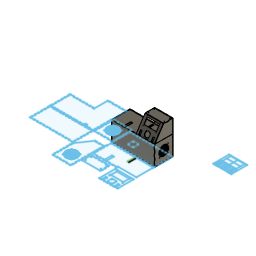
Music Inverntory Machine v29 (1) (Autodesk Fusion 360 design; units mm, degrees)
Autodesk Fusion 360 part; units mm, degrees
note: some values were not read from the file. Set by a fixed rule: which sketch regions a step uses.
(part 1 of 6)
sketch "300mm" plane through (0, 0, 0) normal (0, 0, 1) x (1, 0, 0)
  line L0 (3, 62.25) -> (0, 62.25)
  line L1 (164.25, 6) -> (186.75, 6)
  line L2 (0, 107.25) -> (0, 84.75)
  line L3 (119.25, 6) -> (141.75, 6)
  line L4 (303, 39.75) -> (306, 39.75)
  line L5 (0, 62.25) -> (0, 39.75)
  line L6 (306, 62.25) -> (303, 62.25)
  line L7 (303, 107.25) -> (303, 129.75)
  line L8 (96.75, 6) -> (96.75, 3)
  line L9 (306, 144) -> (276.75, 144)
  line L10 (0, 129.75) -> (3, 129.75)
  line L11 (306, 17.25) -> (303, 17.25)
  line L12 (276.75, 6) -> (276.75, 3)
  line L13 (0, 144) -> (0, 129.75)
  line L14 (51.75, 3) -> (74.25, 3)
  line L15 (231.75, 144) -> (231.75, 141)
  line L16 (74.25, 3) -> (74.25, 6)
  line L17 (306, 39.75) -> (306, 62.25)
  line L18 (231.75, 141) -> (209.25, 141)
  line L19 (0, 39.75) -> (3, 39.75)
  line L20 (186.75, 6) -> (186.75, 3)
  line L21 (96.75, 3) -> (119.25, 3)
  line L22 (74.25, 6) -> (96.75, 6)
  line L23 (254.25, 6) -> (276.75, 6)
  line L24 (0, 17.25) -> (0, 3)
  line L25 (303, 62.25) -> (303, 84.75)
  line L26 (306, 84.75) -> (306, 107.25)
  line L27 (306, 107.25) -> (303, 107.25)
  line L28 (3, 17.25) -> (0, 17.25)
  line L29 (254.25, 3) -> (254.25, 6)
  line L30 (141.75, 3) -> (164.25, 3)
  line L31 (303, 84.75) -> (306, 84.75)
  line L32 (0, 84.75) -> (3, 84.75)
  line L33 (231.75, 6) -> (231.75, 3)
  line L34 (276.75, 3) -> (299.25, 3)
  line L35 (306, 129.75) -> (306, 144)
  line L36 (303, 129.75) -> (306, 129.75)
  line L37 (276.75, 144) -> (276.75, 141)
  line L38 (254.25, 141) -> (254.25, 144)
  line L39 (209.25, 141) -> (209.25, 144)
  line L40 (276.75, 141) -> (254.25, 141)
  line L41 (51.75, 6) -> (51.75, 3)
  line L42 (254.25, 144) -> (231.75, 144)
  line L43 (0, 3) -> (29.25, 3)
  line L44 (231.75, 3) -> (254.25, 3)
  line L45 (3, 107.25) -> (0, 107.25)
  line L46 (209.25, 144) -> (186.75, 144)
  line L47 (209.25, 6) -> (231.75, 6)
  line L48 (29.25, 3) -> (29.25, 6)
  line L49 (3, 129.75) -> (3, 107.25)
  line L50 (141.75, 6) -> (141.75, 3)
  line L51 (299.25, 3) -> (306, 3)
  line L52 (303, 17.25) -> (303, 39.75)
  line L53 (209.25, 3) -> (209.25, 6)
  line L54 (119.25, 3) -> (119.25, 6)
  line L55 (3, 84.75) -> (3, 62.25)
  line L56 (29.25, 6) -> (51.75, 6)
  line L57 (306, 3) -> (306, 17.25)
  line L58 (164.25, 3) -> (164.25, 6)
  line L59 (186.75, 3) -> (209.25, 3)
  line L60 (3, 39.75) -> (3, 17.25)
  line L61 (51.75, 144) -> (51.75, 141)
  line L62 (96.75, 144) -> (96.75, 141)
  line L63 (74.25, 144) -> (51.75, 144)
  line L64 (141.75, 144) -> (141.75, 141)
  line L65 (186.75, 141) -> (164.25, 141)
  line L66 (29.25, 144) -> (6.75, 144)
  line L67 (96.75, 141) -> (74.25, 141)
  line L68 (6.75, 144) -> (0, 144)
  line L69 (74.25, 141) -> (74.25, 144)
  line L70 (164.25, 144) -> (141.75, 144)
  line L71 (119.25, 141) -> (119.25, 144)
  line L72 (141.75, 141) -> (119.25, 141)
  line L73 (119.25, 144) -> (96.75, 144)
  line L74 (51.75, 141) -> (29.25, 141)
  line L75 (186.75, 144) -> (186.75, 141)
  line L76 (164.25, 141) -> (164.25, 144)
  line L77 (29.25, 141) -> (29.25, 144)
  line L78 (441, -20.25) -> (438, -20.25)
  line L79 (441, -42.75) -> (441, -20.25)
  line L80 (408.75, 90.147) -> (408.75, 87.147)
  line L81 (438, -42.75) -> (441, -42.75)
  line L82 (438, -147) -> (438, -132.75)
  line L83 (312, -6) -> (312, -20.25)
  line L84 (438, 90.147) -> (408.75, 90.147)
  line L85 (431.25, -147) -> (438, -147)
  line L86 (309, -87.75) -> (312, -87.75)
  line L87 (312, -42.75) -> (312, -65.25)
  line L88 (312, -87.75) -> (312, -110.25)
  line L89 (441, -132.75) -> (441, -110.25)
  line L90 (309, -42.75) -> (312, -42.75)
  line L91 (312, -65.25) -> (309, -65.25)
  line L92 (438, -20.25) -> (438, 90.147)
  line L93 (363.75, -144) -> (363.75, -147)
  line L94 (408.75, 87.147) -> (386.25, 87.147)
  line L95 (341.25, -144) -> (363.75, -144)
  line L96 (309, -110.25) -> (309, -132.75)
  line L97 (309, -132.75) -> (312, -132.75)
  line L98 (441, -87.75) -> (441, -65.25)
  line L99 (408.75, -147) -> (431.25, -147)
  line L100 (312, -147) -> (341.25, -147)
  line L101 (309, -65.25) -> (309, -87.75)
  line L102 (438, -132.75) -> (441, -132.75)
  line L103 (312, -20.25) -> (309, -20.25)
  line L104 (408.75, -144) -> (408.75, -147)
  line L105 (341.25, -147) -> (341.25, -144)
  line L106 (386.25, 87.147) -> (386.25, 90.147)
  line L107 (312, -132.75) -> (312, -147)
  line L108 (441, -65.25) -> (438, -65.25)
  line L109 (312, -110.25) -> (309, -110.25)
  line L110 (363.75, -147) -> (386.25, -147)
  line L111 (438, -87.75) -> (441, -87.75)
  line L112 (438, -110.25) -> (438, -87.75)
  line L113 (441, -110.25) -> (438, -110.25)
  line L114 (386.25, -147) -> (386.25, -144)
  line L115 (309, -20.25) -> (309, -42.75)
  line L116 (386.25, -144) -> (408.75, -144)
  line L117 (438, -65.25) -> (438, -42.75)
  line L118 (447, 6) -> (473.25, 6)
  line L119 (447, 57.75) -> (444, 57.75)
  line L120 (447, 80.25) -> (447, 57.75)
  line L121 (473.25, 6) -> (473.25, 3)
  line L122 (585.75, 3) -> (585.75, 6)
  line L123 (608.25, 6) -> (608.25, 3)
  line L124 (447, 35.25) -> (447, 12.75)
  line L125 (540.75, 6) -> (563.25, 6)
  line L126 (447, 102.75) -> (444, 102.75)
  line L127 (495.75, 6) -> (518.25, 6)
  line L128 (563.25, 132) -> (540.75, 132)
  line L129 (608.25, 132) -> (585.75, 132)
  line L130 (540.75, 132) -> (540.75, 135)
  line L131 (585.75, 132) -> (585.75, 135)
  line L132 (747, 132) -> (617.8, 132)
  line L133 (747, 125.25) -> (747, 132)
  line L134 (447, 132) -> (447, 102.75)
  line L135 (495.75, 3) -> (495.75, 6)
  line L136 (518.25, 135) -> (518.25, 132)
  line L137 (444, 35.25) -> (447, 35.25)
  line L138 (444, 102.75) -> (444, 80.25)
  line L139 (563.25, 3) -> (585.75, 3)
  line L140 (447, 12.75) -> (447, 6)
  line L141 (563.25, 6) -> (563.25, 3)
  line L142 (518.25, 6) -> (518.25, 3)
  line L143 (585.75, 6) -> (608.25, 6)
  line L144 (540.75, 3) -> (540.75, 6)
  line L145 (608.25, 135) -> (608.25, 132)
  line L146 (473.25, 3) -> (495.75, 3)
  line L147 (747, 12) -> (747, 125.25)
  line L148 (518.25, 3) -> (540.75, 3)
  line L149 (444, 57.75) -> (444, 35.25)
  line L150 (444, 80.25) -> (447, 80.25)
  line L151 (518.25, 132) -> (495.75, 132)
  line L152 (473.25, 132) -> (450.75, 132)
  line L153 (495.75, 132) -> (495.75, 135)
  line L154 (473.25, 135) -> (473.25, 132)
  line L155 (563.25, 135) -> (563.25, 132)
  line L156 (450.75, 132) -> (447, 132)
  line L157 (540.75, 135) -> (518.25, 135)
  line L158 (585.75, 135) -> (563.25, 135)
  line L159 (495.75, 135) -> (473.25, 135)
  line L160 (29.25, 150) -> (51.75, 150)
  line L161 (51.75, 150) -> (51.75, 147)
  line L162 (276.75, 150) -> (276.75, 147)
  line L163 (0, 161.25) -> (0, 147)
  line L164 (29.25, 147) -> (29.25, 150)
  line L165 (96.75, 147) -> (119.25, 147)
  line L166 (51.75, 147) -> (74.25, 147)
  line L167 (3, 206.25) -> (0, 206.25)
  line L168 (209.25, 147) -> (209.25, 150)
  line L169 (119.25, 147) -> (119.25, 150)
  line L170 (3, 251.25) -> (0, 251.25)
  line L171 (231.75, 147) -> (254.25, 147)
  line L172 (209.25, 150) -> (231.75, 150)
  line L173 (3, 161.25) -> (0, 161.25)
  line L174 (231.75, 150) -> (231.75, 147)
  line L175 (0, 206.25) -> (0, 183.75)
  line L176 (254.25, 147) -> (254.25, 150)
  line L177 (0, 183.75) -> (3, 183.75)
  line L178 (3, 273.75) -> (3, 251.25)
  line L179 (74.25, 147) -> (74.25, 150)
  line L180 (0, 147) -> (29.25, 147)
  line L181 (119.25, 150) -> (141.75, 150)
  line L182 (164.25, 147) -> (164.25, 150)
  line L183 (3, 228.75) -> (3, 206.25)
  line L184 (164.25, 150) -> (186.75, 150)
  line L185 (186.75, 147) -> (209.25, 147)
  line L186 (0, 273.75) -> (3, 273.75)
  line L187 (303, 206.25) -> (303, 228.75)
  line L188 (141.75, 150) -> (141.75, 147)
  line L189 (306, 206.25) -> (303, 206.25)
  line L190 (96.75, 150) -> (96.75, 147)
  line L191 (276.75, 384.147) -> (276.75, 381.147)
  line L192 (299.25, 147) -> (306, 147)
  line L193 (141.75, 147) -> (164.25, 147)
  line L194 (0, 228.75) -> (3, 228.75)
  line L195 (0, 288) -> (0, 273.75)
  line L196 (74.25, 150) -> (96.75, 150)
  line L197 (186.75, 150) -> (186.75, 147)
  line L198 (254.25, 150) -> (276.75, 150)
  line L199 (276.75, 147) -> (299.25, 147)
  line L200 (0, 251.25) -> (0, 228.75)
  line L201 (3, 183.75) -> (3, 161.25)
  line L202 (231.75, 381.147) -> (209.25, 381.147)
  line L203 (164.25, 288) -> (141.75, 288)
  line L204 (306, 273.75) -> (306, 384.147)
  line L205 (96.75, 288) -> (96.75, 285)
  line L206 (51.75, 285) -> (29.25, 285)
  line L207 (303, 251.25) -> (303, 273.75)
  line L208 (141.75, 285) -> (119.25, 285)
  line L209 (186.75, 384.147) -> (186.75, 381.147)
  line L210 (306, 183.75) -> (306, 206.25)
  line L211 (306, 384.147) -> (276.75, 384.147)
  line L212 (141.75, 288) -> (141.75, 285)
  line L213 (254.25, 381.147) -> (254.25, 384.147)
  line L214 (276.75, 381.147) -> (254.25, 381.147)
  line L215 (254.25, 384.147) -> (231.75, 384.147)
  line L216 (6.75, 288) -> (0, 288)
  line L217 (231.75, 384.147) -> (231.75, 381.147)
  line L218 (306, 228.75) -> (306, 251.25)
  line L219 (303, 228.75) -> (306, 228.75)
  line L220 (29.25, 288) -> (6.75, 288)
  line L221 (29.25, 285) -> (29.25, 288)
  line L222 (164.25, 285) -> (164.25, 288)
  line L223 (96.75, 285) -> (74.25, 285)
  line L224 (119.25, 285) -> (119.25, 288)
  line L225 (306, 251.25) -> (303, 251.25)
  line L226 (119.25, 288) -> (96.75, 288)
  line L227 (74.25, 288) -> (51.75, 288)
  line L228 (209.25, 384.147) -> (186.75, 384.147)
  line L229 (306, 161.25) -> (303, 161.25)
  line L230 (209.25, 381.147) -> (209.25, 384.147)
  line L231 (303, 161.25) -> (303, 183.75)
  line L232 (303, 273.75) -> (306, 273.75)
  line L233 (173.8, 285) -> (164.25, 285)
  line L234 (303, 183.75) -> (306, 183.75)
  line L235 (306, 147) -> (306, 161.25)
  line L236 (51.75, 288) -> (51.75, 285)
  line L237 (74.25, 285) -> (74.25, 288)
  line L238 (309, 161.25) -> (312, 161.25)
  line L239 (386.25, 285) -> (386.25, 288)
  line L240 (312, 206.25) -> (312, 183.75)
  line L241 (309, 228.75) -> (309, 206.25)
  line L242 (309, 183.75) -> (309, 161.25)
  line L243 (341.25, 150) -> (363.75, 150)
  line L244 (386.25, 147) -> (386.25, 150)
  line L245 (441, 183.75) -> (438, 183.75)
  line L246 (341.25, 285) -> (341.25, 288)
  line L247 (438, 288) -> (408.75, 288)
  line L248 (341.25, 288) -> (318.75, 288)
  line L249 (438, 228.75) -> (438, 251.25)
  line L250 (386.25, 150) -> (408.75, 150)
  line L251 (312, 251.25) -> (312, 228.75)
  line L252 (309, 273.75) -> (309, 251.25)
  line L253 (309, 206.25) -> (312, 206.25)
  line L254 (438, 183.75) -> (438, 206.25)
  line L255 (408.75, 288) -> (408.75, 285)
  line L256 (438, 273.75) -> (438, 288)
  line L257 (363.75, 285) -> (341.25, 285)
  line L258 (312, 183.75) -> (309, 183.75)
  line L259 (312, 228.75) -> (309, 228.75)
  line L260 (312, 161.25) -> (312, 147)
  line L261 (309, 251.25) -> (312, 251.25)
  line L262 (408.75, 285) -> (386.25, 285)
  line L263 (312, 273.75) -> (309, 273.75)
  line L264 (363.75, 147) -> (386.25, 147)
  line L265 (318.75, 288) -> (312, 288)
  line L266 (363.75, 288) -> (363.75, 285)
  line L267 (441, 251.25) -> (441, 273.75)
  line L268 (441, 161.25) -> (441, 183.75)
  line L269 (386.25, 288) -> (363.75, 288)
  line L270 (341.25, 147) -> (341.25, 150)
  line L271 (438, 206.25) -> (441, 206.25)
  line L272 (438, 147) -> (438, 161.25)
  line L273 (431.25, 147) -> (438, 147)
  line L274 (438, 251.25) -> (441, 251.25)
  line L275 (438, 161.25) -> (441, 161.25)
  line L276 (312, 147) -> (341.25, 147)
  line L277 (363.75, 150) -> (363.75, 147)
  line L278 (408.75, 150) -> (408.75, 147)
  line L279 (441, 273.75) -> (438, 273.75)
  line L280 (312, 288) -> (312, 273.75)
  line L281 (408.75, 147) -> (431.25, 147)
  line L282 (441, 206.25) -> (441, 228.75)
  line L283 (441, 228.75) -> (438, 228.75)
  line L284 (447, 141) -> (473.25, 141)
  line L285 (585.75, 138) -> (585.75, 141)
  line L286 (698.25, 141) -> (698.25, 138)
  line L287 (447, 192.75) -> (444, 192.75)
  line L288 (608.25, 141) -> (608.25, 138)
  line L289 (447, 267) -> (447, 237.75)
  line L290 (444, 170.25) -> (447, 170.25)
  line L291 (495.75, 138) -> (495.75, 141)
  line L292 (585.75, 141) -> (608.25, 141)
  line L293 (747, 170.25) -> (750, 170.25)
  line L294 (675.75, 141) -> (698.25, 141)
  line L295 (750, 170.25) -> (750, 192.75)
  line L296 (743.25, 141) -> (747, 141)
  line L297 (608.25, 138) -> (630.75, 138)
  line L298 (447, 147.75) -> (447, 141)
  line L299 (747, 141) -> (747, 170.25)
  line L300 (630.75, 141) -> (653.25, 141)
  line L301 (563.25, 138) -> (585.75, 138)
  line L302 (447, 215.25) -> (447, 192.75)
  line L303 (675.75, 138) -> (675.75, 141)
  line L304 (518.25, 138) -> (540.75, 138)
  line L305 (495.75, 141) -> (518.25, 141)
  line L306 (653.25, 141) -> (653.25, 138)
  line L307 (447, 170.25) -> (447, 147.75)
  line L308 (698.25, 138) -> (720.75, 138)
  line L309 (444, 215.25) -> (447, 215.25)
  line L310 (447, 237.75) -> (444, 237.75)
  line L311 (540.75, 138) -> (540.75, 141)
  line L312 (630.75, 138) -> (630.75, 141)
  line L313 (653.25, 138) -> (675.75, 138)
  line L314 (720.75, 138) -> (720.75, 141)
  line L315 (518.25, 141) -> (518.25, 138)
  line L316 (720.75, 141) -> (743.25, 141)
  line L317 (444, 192.75) -> (444, 170.25)
  line L318 (608.25, 270) -> (608.25, 267)
  line L319 (720.75, 270) -> (698.25, 270)
  line L320 (630.75, 270) -> (608.25, 270)
  line L321 (563.25, 267) -> (540.75, 267)
  line L322 (747, 267) -> (720.75, 267)
  line L323 (747, 237.75) -> (747, 260.25)
  line L324 (675.75, 267) -> (675.75, 270)
  line L325 (495.75, 270) -> (473.25, 270)
  line L326 (585.75, 267) -> (585.75, 270)
  line L327 (630.75, 267) -> (630.75, 270)
  line L328 (750, 215.25) -> (750, 237.75)
  line L329 (747, 260.25) -> (747, 267)
  line L330 (720.75, 267) -> (720.75, 270)
  line L331 (518.25, 270) -> (518.25, 267)
  line L332 (540.75, 270) -> (518.25, 270)
  line L333 (747, 215.25) -> (750, 215.25)
  line L334 (675.75, 270) -> (653.25, 270)
  line L335 (750, 192.75) -> (747, 192.75)
  line L336 (698.25, 270) -> (698.25, 267)
  line L337 (473.25, 141) -> (473.25, 138)
  line L338 (495.75, 267) -> (495.75, 270)
  line L339 (540.75, 267) -> (540.75, 270)
  line L340 (540.75, 141) -> (563.25, 141)
  line L341 (563.25, 270) -> (563.25, 267)
  line L342 (653.25, 267) -> (630.75, 267)
  line L343 (747, 192.75) -> (747, 215.25)
  line L344 (563.25, 141) -> (563.25, 138)
  line L345 (473.25, 267) -> (450.75, 267)
  line L346 (750, 237.75) -> (747, 237.75)
  line L347 (698.25, 267) -> (675.75, 267)
  line L348 (585.75, 270) -> (563.25, 270)
  line L349 (450.75, 267) -> (447, 267)
  line L350 (653.25, 270) -> (653.25, 267)
  line L351 (473.25, 138) -> (495.75, 138)
  line L352 (608.25, 267) -> (585.75, 267)
  line L353 (518.25, 267) -> (495.75, 267)
  line L354 (473.25, 270) -> (473.25, 267)
  line L355 (444, 237.75) -> (444, 215.25)
  line L356 (396.25, 205.4178) -> (394.25, 206.5725)
  line L357 (397.75, 203.1084) -> (399.75, 201.9537)
  line L358 (401.75, 203.1084) -> (401.75, 205.4178)
  line L359 (399, 200.6547) -> (397, 201.8094)
  line L360 (396.25, 203.1084) -> (396.25, 205.4178)
  line L361 (401.75, 205.4178) -> (399.75, 206.5725)
  line L362 (395, 198.3453) -> (397, 197.1906)
  line L363 (401.75, 196.4178) -> (399.75, 197.5725)
  line L364 (397.75, 196.4178) -> (397.75, 194.1084)
  line L365 (397.75, 196.4178) -> (397.75, 194.1084)
  arc A0 (400.2057, 193.2169) -> (401.75, 194.9293) centre (375, 217.5) ccw
  line L366 (397, 197.1906) -> (399, 198.3453)
  line L367 (397.75, 194.1084) -> (399.75, 192.9537)
  line L368 (396.25, 196.4178) -> (394.25, 197.5725)
  line L369 (396.25, 196.4178) -> (394.25, 197.5725)
  line L370 (401.75, 194.9293) -> (401.75, 196.4178)
  line L371 (399.75, 192.9537) -> (400.2057, 193.2169)
  arc A1 (400.2057, 193.2169) -> (401.75, 194.9293) centre (375, 217.5) ccw
  line L372 (396.25, 194.1084) -> (396.25, 196.4178)
  line L373 (396.25, 194.1084) -> (396.25, 196.4178)
  line L374 (401.75, 196.4178) -> (399.75, 197.5725)
  line L375 (397.75, 194.1084) -> (399.75, 192.9537)
  line L376 (399.75, 192.9537) -> (400.2057, 193.2169)
  line L377 (399.75, 197.5725) -> (397.75, 196.4178)
  line L378 (401.75, 194.9293) -> (401.75, 196.4178)
  line L379 (395, 198.3453) -> (397, 197.1906)
  line L380 (399.75, 197.5725) -> (397.75, 196.4178)
  line L381 (397, 197.1906) -> (399, 198.3453)
  line L382 (394.25, 192.9537) -> (396.25, 194.1084)
  line L383 (394.25, 192.9537) -> (396.25, 194.1084)
  line L384 (375, 188.1906) -> (377, 189.3453)
  line L385 (389.5, 191.6547) -> (389.5, 189.3453)
  arc A2 (395.442, 189.0901) -> (398.7552, 191.7961) centre (375, 217.5) ccw
  line L386 (395, 189.3453) -> (395.442, 189.0901)
  line L387 (395, 191.6547) -> (395, 189.3453)
  arc A3 (395.442, 189.0901) -> (398.7552, 191.7961) centre (375, 217.5) ccw
  line L388 (395, 191.6547) -> (395, 189.3453)
  line L389 (395, 189.3453) -> (395.442, 189.0901)
  line L390 (396.25, 212.1084) -> (396.25, 214.4178)
  line L391 (397.75, 214.4178) -> (397.75, 212.1084)
  line L392 (377, 236.6547) -> (375, 237.8094)
  line L393 (395, 216.3453) -> (397, 215.1906)
  line L394 (399.75, 210.9537) -> (401.75, 212.1084)
  line L395 (375, 206.1906) -> (377, 207.3453)
  line L396 (399, 209.6547) -> (397, 210.8094)
  line L397 (397.75, 212.1084) -> (399.75, 210.9537)
  line L398 (399, 209.6547) -> (397, 210.8094)
  line L399 (397.75, 212.1084) -> (399.75, 210.9537)
  line L400 (396.25, 214.4178) -> (394.25, 215.5725)
  line L401 (375, 197.1906) -> (377, 198.3453)
  line L402 (397.75, 214.4178) -> (397.75, 212.1084)
  line L403 (375, 206.1906) -> (377, 207.3453)
  line L404 (401.75, 212.1084) -> (401.75, 214.4178)
  line L405 (375, 224.1906) -> (377, 225.3453)
  line L406 (394.25, 210.9537) -> (396.25, 212.1084)
  arc A4 (377, 252.4428) -> (373, 252.4428) centre (375, 217.5) ccw
  line L407 (375, 215.1906) -> (377, 216.3453)
  line L408 (377, 209.6547) -> (375, 210.8094)
  line L409 (375, 233.1906) -> (377, 234.3453)
  line L410 (399.75, 210.9537) -> (401.75, 212.1084)
  line L411 (377, 182.6547) -> (375, 183.8094)
  line L412 (375, 215.1906) -> (377, 216.3453)
  line L413 (375, 251.1906) -> (377, 252.3453)
  line L414 (401.75, 214.4178) -> (399.75, 215.5725)
  line L415 (395, 216.3453) -> (397, 215.1906)
  line L416 (377, 245.6547) -> (375, 246.8094)
  line L417 (401.75, 214.4178) -> (399.75, 215.5725)
  line L418 (396.25, 214.4178) -> (394.25, 215.5725)
  line L419 (396.25, 212.1084) -> (396.25, 214.4178)
  line L420 (375, 188.1906) -> (377, 189.3453)
  line L421 (375, 224.1906) -> (377, 225.3453)
  line L422 (377, 200.6547) -> (375, 201.8094)
  line L423 (375, 251.1906) -> (377, 252.3453)
  line L424 (397, 215.1906) -> (399, 216.3453)
  line L425 (377, 191.6547) -> (375, 192.8094)
  line L426 (377, 182.6547) -> (375, 183.8094)
  line L427 (377, 236.6547) -> (375, 237.8094)
  line L428 (397, 210.8094) -> (395, 209.6547)
  line L429 (377, 227.6547) -> (375, 228.8094)
  line L430 (375, 197.1906) -> (377, 198.3453)
  line L431 (377, 200.6547) -> (375, 201.8094)
  line L432 (377, 209.6547) -> (375, 210.8094)
  line L433 (398.7552, 191.7961) -> (397, 192.8094)
  line L434 (377, 191.6547) -> (375, 192.8094)
  line L435 (401.75, 223.4178) -> (399.75, 224.5725)
  line L436 (394.25, 197.5725) -> (392.25, 196.4178)
  arc A5 (342.75, 203.9008) -> (343.2193, 202.8375) centre (375, 217.5) ccw
  line L437 (391.5, 215.1906) -> (393.5, 216.3453)
  line L438 (348.25, 205.4178) -> (348.25, 203.1084)
  line L439 (386, 192.8094) -> (384, 191.6547)
  line L440 (368.75, 203.1084) -> (368.75, 205.4178)
  line L441 (375, 242.1906) -> (377, 243.3453)
  line L442 (353.75, 205.4178) -> (353.75, 203.1084)
  line L443 (377, 227.6547) -> (375, 228.8094)
  line L444 (399.75, 215.5725) -> (397.75, 214.4178)
  line L445 (380.5, 192.8094) -> (378.5, 191.6547)
  line L446 (377, 218.6547) -> (375, 219.8094)
  line L447 (397, 215.1906) -> (399, 216.3453)
  line L448 (346.75, 203.1084) -> (346.75, 205.4178)
  line L449 (386, 192.8094) -> (384, 191.6547)
  line L450 (382.5, 191.6547) -> (380.5, 192.8094)
  line L451 (399.75, 215.5725) -> (397.75, 214.4178)
  line L452 (391.5, 192.8094) -> (389.5, 191.6547)
  arc A6 (342.75, 203.9008) -> (343.2193, 202.8375) centre (375, 217.5) ccw
  line L453 (363.25, 203.1084) -> (363.25, 205.4178)
  line L454 (348.25, 205.4178) -> (348.25, 203.1084)
  line L455 (359.25, 205.4178) -> (359.25, 203.1084)
  line L456 (394.25, 210.9537) -> (396.25, 212.1084)
  line L457 (353.75, 205.4178) -> (353.75, 203.1084)
  line L458 (397, 192.8094) -> (395, 191.6547)
  line L459 (377, 245.6547) -> (375, 246.8094)
  line L460 (352.25, 203.1084) -> (352.25, 205.4178)
  line L461 (393.5, 191.6547) -> (391.5, 192.8094)
  line L462 (391.5, 192.8094) -> (389.5, 191.6547)
  line L463 (382.5, 191.6547) -> (380.5, 192.8094)
  line L464 (395, 225.3453) -> (397, 224.1906)
  line L465 (399, 218.6547) -> (397, 219.8094)
  line L466 (398.7552, 191.7961) -> (397, 192.8094)
  line L467 (397, 210.8094) -> (395, 209.6547)
  line L468 (388, 191.6547) -> (386, 192.8094)
  line L469 (401.75, 212.1084) -> (401.75, 214.4178)
  line L470 (380.5, 192.8094) -> (378.5, 191.6547)
  arc A7 (373, 182.5572) -> (377, 182.5572) centre (375, 217.5) ccw
  line L471 (396.25, 221.1084) -> (396.25, 223.4178)
  line L472 (357.75, 203.1084) -> (357.75, 205.4178)
  line L473 (377, 218.6547) -> (375, 219.8094)
  line L474 (357.75, 203.1084) -> (357.75, 205.4178)
  line L475 (397, 192.8094) -> (395, 191.6547)
  line L476 (346.75, 203.1084) -> (346.75, 205.4178)
  line L477 (399, 218.6547) -> (397, 219.8094)
  line L478 (374.25, 203.1084) -> (374.25, 205.4178)
  line L479 (397, 219.8094) -> (395, 218.6547)
  line L480 (370.25, 205.4178) -> (370.25, 203.1084)
  line L481 (364.75, 205.4178) -> (364.75, 203.1084)
  line L482 (396.25, 221.1084) -> (396.25, 223.4178)
  line L483 (359.25, 205.4178) -> (359.25, 203.1084)
  arc A8 (373, 182.5572) -> (377, 182.5572) centre (375, 217.5) ccw
  line L484 (393.5, 191.6547) -> (391.5, 192.8094)
  line L485 (388, 191.6547) -> (386, 192.8094)
  line L486 (352.25, 203.1084) -> (352.25, 205.4178)
  line L487 (364.75, 205.4178) -> (364.75, 203.1084)
  line L488 (368.75, 203.1084) -> (368.75, 205.4178)
  line L489 (397.75, 223.4178) -> (397.75, 221.1084)
  line L490 (363.25, 203.1084) -> (363.25, 205.4178)
  line L491 (401.75, 223.4178) -> (399.75, 224.5725)
  line L492 (394.25, 219.9537) -> (396.25, 221.1084)
  line L493 (363.25, 187.4178) -> (361.25, 188.5725)
  line L494 (359.25, 194.1084) -> (361.25, 192.9537)
  line L495 (361.25, 197.5725) -> (359.25, 196.4178)
  line L496 (392.25, 203.1084) -> (394.25, 201.9537)
  line L497 (344.75, 201.9537) -> (346.75, 203.1084)
  line L498 (370.25, 205.4178) -> (370.25, 203.1084)
  line L499 (347.5, 197.1906) -> (349.5, 198.3453)
  line L500 (344.75, 215.5725) -> (342.75, 214.4178)
  line L501 (391.5, 206.1906) -> (393.5, 207.3453)
  line L502 (347.5, 197.1906) -> (349.5, 198.3453)
  line L503 (392.25, 239.1084) -> (394.25, 237.9537)
  line L504 (392.25, 221.1084) -> (394.25, 219.9537)
  line L505 (394.25, 215.5725) -> (392.25, 214.4178)
  line L506 (347.5, 201.8094) -> (345.5, 200.6547)
  line L507 (349.5, 200.6547) -> (347.5, 201.8094)
  line L508 (374.25, 203.1084) -> (374.25, 205.4178)
  line L509 (344.75, 233.5725) -> (343.5641, 232.8879)
  line L510 (392.25, 203.1084) -> (394.25, 201.9537)
  line L511 (342.75, 212.1084) -> (344.75, 210.9537)
  line L512 (342.75, 221.1084) -> (344.75, 219.9537)
  line L513 (344.75, 206.5725) -> (342.75, 205.4178)
  line L514 (401.75, 221.1084) -> (401.75, 223.4178)
  line L515 (393.5, 209.6547) -> (391.5, 210.8094)
  line L516 (344.75, 224.5725) -> (342.75, 223.4178)
  line L517 (397, 224.1906) -> (399, 225.3453)
  line L518 (399.75, 224.5725) -> (397.75, 223.4178)
  line L519 (397.75, 223.4178) -> (397.75, 221.1084)
  line L520 (391.5, 233.1906) -> (393.5, 234.3453)
  line L521 (345.8335, 198.1527) -> (347.5, 197.1906)
  line L522 (345.8335, 198.1527) -> (347.5, 197.1906)
  line L523 (391.5, 242.1906) -> (393.5, 243.3453)
  line L524 (391.5, 224.1906) -> (393.5, 225.3453)
  line L525 (399.75, 219.9537) -> (401.75, 221.1084)
  line L526 (391.5, 224.1906) -> (393.5, 225.3453)
  line L527 (392.25, 221.1084) -> (394.25, 219.9537)
  line L528 (342.75, 230.1084) -> (344.75, 228.9537)
  line L529 (396.25, 223.4178) -> (394.25, 224.5725)
  line L530 (393.5, 200.6547) -> (391.5, 201.8094)
  line L531 (342.75, 212.1084) -> (344.75, 210.9537)
  line L532 (347.5, 201.8094) -> (345.5, 200.6547)
  line L533 (397, 219.8094) -> (395, 218.6547)
  line L534 (397.75, 221.1084) -> (399.75, 219.9537)
  line L535 (396.25, 223.4178) -> (394.25, 224.5725)
  line L536 (391.5, 233.1906) -> (393.5, 234.3453)
  line L537 (344.75, 215.5725) -> (342.75, 214.4178)
  line L538 (397.75, 221.1084) -> (399.75, 219.9537)
  line L539 (344.75, 206.5725) -> (342.75, 205.4178)
  line L540 (394.25, 219.9537) -> (396.25, 221.1084)
  line L541 (344.75, 224.5725) -> (342.75, 223.4178)
  line L542 (349.5, 200.6547) -> (347.5, 201.8094)
  line L543 (342.75, 230.1084) -> (344.75, 228.9537)
  line L544 (393.5, 209.6547) -> (391.5, 210.8094)
  line L545 (395, 225.3453) -> (397, 224.1906)
  line L546 (394.25, 242.5725) -> (392.25, 241.4178)
  line L547 (401.75, 221.1084) -> (401.75, 223.4178)
  line L548 (393.5, 245.6547) -> (391.5, 246.8094)
  line L549 (393.5, 216.3453) -> (393.5, 218.6547)
  line L550 (399, 216.3453) -> (399, 218.6547)
  line L551 (363.25, 214.4178) -> (361.25, 215.5725)
  line L552 (370.25, 187.4178) -> (370.25, 185.1084)
  line L553 (399.75, 219.9537) -> (401.75, 221.1084)
  line L554 (374.25, 205.4178) -> (372.25, 206.5725)
  line L555 (341.8476, 206.2786) -> (342, 206.1906)
  line L556 (361.25, 188.5725) -> (359.25, 187.4178)
  line L557 (361.25, 201.9537) -> (363.25, 203.1084)
  line L558 (363.25, 187.4178) -> (361.25, 188.5725)
  line L559 (343.2193, 202.8375) -> (344.75, 201.9537)
  line L560 (393.5, 216.3453) -> (393.5, 218.6547)
  line L561 (361.25, 192.9537) -> (363.25, 194.1084)
  line L562 (374.25, 187.4178) -> (372.25, 188.5725)
  line L563 (361.25, 246.9537) -> (363.25, 248.1084)
  line L564 (399, 216.3453) -> (399, 218.6547)
  line L565 (361.25, 210.9537) -> (363.25, 212.1084)
  line L566 (345.5, 200.6547) -> (345.5, 198.6652)
  arc A9 (345.5, 198.6652) -> (345.8335, 198.1527) centre (375, 217.5) ccw
  line L567 (341.25, 221.1084) -> (341.25, 223.4178)
  line L568 (373, 182.6547) -> (373, 182.5572)
  line L569 (395, 218.6547) -> (395, 216.3453)
  line L570 (370.25, 187.4178) -> (370.25, 185.1084)
  line L571 (343.2193, 202.8375) -> (344.75, 201.9537)
  line L572 (372.25, 188.5725) -> (370.25, 187.4178)
  line L573 (400.5, 216.3453) -> (402.5, 215.1906)
  line L574 (344.75, 201.9537) -> (346.75, 203.1084)
  line L575 (345.5, 200.6547) -> (345.5, 198.6652)
  line L576 (397, 224.1906) -> (399, 225.3453)
  line L577 (342.75, 221.1084) -> (344.75, 219.9537)
  line L578 (394.25, 206.5725) -> (392.25, 205.4178)
  line L579 (373, 189.3453) -> (375, 188.1906)
  line L580 (341.25, 221.1084) -> (341.25, 223.4178)
  line L581 (375, 183.8094) -> (373, 182.6547)
  line L582 (400.5, 218.6547) -> (400.5, 216.3453)
  line L583 (402.5, 210.8094) -> (400.5, 209.6547)
  line L584 (342.75, 223.4178) -> (342.75, 221.1084)
  line L585 (392.25, 194.1084) -> (394.25, 192.9537)
  line L586 (373, 189.3453) -> (375, 188.1906)
  line L587 (344.75, 233.5725) -> (343.5641, 232.8879)
  line L588 (395, 218.6547) -> (395, 216.3453)
  arc A10 (340.5732, 223.8086) -> (340.1253, 220.4591) centre (375, 217.5) ccw
  line L589 (361.25, 197.5725) -> (359.25, 196.4178)
  line L590 (400.5, 225.3453) -> (402.5, 224.1906)
  line L591 (394.25, 224.5725) -> (392.25, 223.4178)
  line L592 (371.5, 209.6547) -> (369.5, 210.8094)
  line L593 (363.25, 196.4178) -> (361.25, 197.5725)
  line L594 (394.25, 206.5725) -> (392.25, 205.4178)
  line L595 (393.5, 245.6547) -> (391.5, 246.8094)
  line L596 (399.75, 224.5725) -> (397.75, 223.4178)
  line L597 (342.75, 223.4178) -> (342.75, 221.1084)
  line L598 (393.5, 218.6547) -> (391.5, 219.8094)
  arc A11 (345.5, 198.6652) -> (345.8335, 198.1527) centre (375, 217.5) ccw
  line L599 (400.5, 218.6547) -> (400.5, 216.3453)
  line L600 (394.25, 224.5725) -> (392.25, 223.4178)
  arc A12 (340.5732, 223.8086) -> (340.1253, 220.4591) centre (375, 217.5) ccw
  line L601 (361.25, 237.9537) -> (363.25, 239.1084)
  arc A13 (359.25, 186.244) -> (362.6388, 184.7555) centre (375, 217.5) ccw
  line L602 (342, 210.8094) -> (340.789, 210.1102)
  line L603 (404.5, 209.6547) -> (402.5, 210.8094)
  line L604 (394.25, 233.5725) -> (392.25, 232.4178)
  line L605 (344, 209.6547) -> (342, 210.8094)
  line L606 (342, 224.1906) -> (344, 225.3453)
  line L607 (341.8476, 206.2786) -> (342, 206.1906)
  line L608 (363.25, 205.4178) -> (361.25, 206.5725)
  line L609 (342, 206.1906) -> (344, 207.3453)
  line L610 (402.5, 215.1906) -> (404.5, 216.3453)
  line L611 (402.5, 224.1906) -> (404.5, 225.3453)
  line L612 (374.25, 205.4178) -> (372.25, 206.5725)
  line L613 (372.25, 183.9537) -> (374.25, 185.1084)
  line L614 (370.25, 185.1084) -> (372.25, 183.9537)
  line L615 (340.4891, 211.6691) -> (341.25, 212.1084)
  line L616 (342.75, 205.4178) -> (342.75, 203.9008)
  line L617 (375, 183.8094) -> (373, 182.6547)
  line L618 (362, 234.3453) -> (364, 233.1906)
  line L619 (342, 210.8094) -> (340.789, 210.1102)
  line L620 (402.5, 210.8094) -> (400.5, 209.6547)
  line L621 (341.25, 223.4178) -> (340.5732, 223.8086)
  line L622 (371.5, 209.6547) -> (369.5, 210.8094)
  line L623 (342.75, 231.0992) -> (342.75, 230.1084)
  line L624 (342, 206.1906) -> (344, 207.3453)
  line L625 (402.5, 215.1906) -> (404.5, 216.3453)
  line L626 (372.25, 188.5725) -> (370.25, 187.4178)
  line L627 (392.25, 230.1084) -> (394.25, 228.9537)
  line L628 (370.25, 212.1084) -> (372.25, 210.9537)
  line L629 (370.25, 212.1084) -> (372.25, 210.9537)
  arc A14 (343.5641, 232.8879) -> (342.75, 231.0992) centre (375, 217.5) ccw
  line L630 (363.25, 241.4178) -> (361.25, 242.5725)
  line L631 (404.5, 218.6547) -> (402.5, 219.8094)
  line L632 (373, 207.3453) -> (375, 206.1906)
  line L633 (372.25, 183.9537) -> (374.25, 185.1084)
  line L634 (370.25, 185.1084) -> (372.25, 183.9537)
  line L635 (402.5, 219.8094) -> (400.5, 218.6547)
  line L636 (361.25, 188.5725) -> (359.25, 187.4178)
  line L637 (344, 225.3453) -> (344, 227.6547)
  arc A15 (343.5641, 232.8879) -> (342.75, 231.0992) centre (375, 217.5) ccw
  line L638 (402.5, 224.1906) -> (404.5, 225.3453)
  line L639 (342.75, 231.0992) -> (342.75, 230.1084)
  line L640 (371.5, 207.3453) -> (371.5, 209.6547)
  line L641 (359.25, 203.1084) -> (361.25, 201.9537)
  line L642 (402.5, 219.8094) -> (400.5, 218.6547)
  line L643 (372.25, 210.9537) -> (374.25, 212.1084)
  line L644 (340.789, 224.8898) -> (342, 224.1906)
  arc A16 (340.789, 210.1102) -> (341.8476, 206.2786) centre (375, 217.5) ccw
  line L645 (374.25, 187.4178) -> (372.25, 188.5725)
  line L646 (340.4891, 211.6691) -> (341.25, 212.1084)
  line L647 (393.5, 200.6547) -> (391.5, 201.8094)
  line L648 (373, 182.6547) -> (373, 182.5572)
  line L649 (373, 207.3453) -> (375, 206.1906)
  line L650 (342, 224.1906) -> (344, 225.3453)
  line L651 (400.5, 225.3453) -> (402.5, 224.1906)
  line L652 (374.25, 185.1084) -> (374.25, 187.4178)
  line L653 (371.5, 207.3453) -> (371.5, 209.6547)
  line L654 (392.25, 239.1084) -> (394.25, 237.9537)
  line L655 (391.5, 197.1906) -> (393.5, 198.3453)
  line L656 (404.5, 218.6547) -> (402.5, 219.8094)
  line L657 (372.25, 210.9537) -> (374.25, 212.1084)
  line L658 (344, 225.3453) -> (344, 227.6547)
  line L659 (374.25, 185.1084) -> (374.25, 187.4178)
  line L660 (400.5, 216.3453) -> (402.5, 215.1906)
  line L661 (369.5, 206.1906) -> (371.5, 207.3453)
  line L662 (342.75, 205.4178) -> (342.75, 203.9008)
  line L663 (344, 227.6547) -> (342, 228.8094)
  line L664 (344, 207.3453) -> (344, 209.6547)
  line L665 (391.5, 197.1906) -> (393.5, 198.3453)
  line L666 (372.25, 206.5725) -> (370.25, 205.4178)
  line L667 (375, 210.8094) -> (373, 209.6547)
  line L668 (404.5, 209.6547) -> (402.5, 210.8094)
  line L669 (364, 219.8094) -> (362, 218.6547)
  line L670 (344, 207.3453) -> (344, 209.6547)
  line L671 (344, 227.6547) -> (342, 228.8094)
  line L672 (404.5, 207.3453) -> (404.5, 209.6547)
  line L673 (353, 237.8094) -> (351, 236.6547)
  line L674 (350.25, 228.9537) -> (352.25, 230.1084)
  line L675 (363.25, 248.1084) -> (363.25, 250.4178)
  line L676 (360.5, 243.3453) -> (360.5, 245.6547)
  line L677 (383.25, 233.5725) -> (381.25, 232.4178)
  line L678 (352.25, 230.1084) -> (352.25, 232.4178)
  line L679 (346.75, 223.4178) -> (344.75, 224.5725)
  line L680 (364.75, 248.1084) -> (366.75, 246.9537)
  line L681 (356.5, 243.3453) -> (358.5, 242.1906)
  line L682 (353, 224.1906) -> (355, 225.3453)
  line L683 (380.5, 237.8094) -> (378.5, 236.6547)
  line L684 (357.75, 241.4178) -> (355.75, 242.5725)
  line L685 (352.25, 230.1084) -> (352.25, 232.4178)
  line L686 (381.25, 239.1084) -> (383.25, 237.9537)
  line L687 (364.75, 250.4178) -> (364.75, 248.1084)
  line L688 (359.25, 248.1084) -> (361.25, 246.9537)
  line L689 (366, 245.6547) -> (364, 246.8094)
  line L690 (344.75, 228.9537) -> (346.75, 230.1084)
  line L691 (347.5, 224.1906) -> (349.5, 225.3453)
  line L692 (346.75, 230.1084) -> (346.75, 232.4178)
  line L693 (383.25, 237.9537) -> (385.25, 239.1084)
  line L694 (369.5, 246.8094) -> (367.5, 245.6547)
  line L695 (363.25, 250.4178) -> (363.1955, 250.4493)
  line L696 (358.5, 246.8094) -> (356.5, 245.6547)
  line L697 (348.25, 230.1084) -> (350.25, 228.9537)
  line L698 (366.573, 251.4704) -> (364.75, 250.4178)
  line L699 (381.25, 239.1084) -> (383.25, 237.9537)
  line L700 (353, 228.8094) -> (351, 227.6547)
  line L701 (368.75, 250.4178) -> (366.8218, 251.5311)
  line L702 (366.75, 246.9537) -> (368.75, 248.1084)
  line L703 (378.5, 234.3453) -> (380.5, 233.1906)
  line L704 (378.5, 234.3453) -> (380.5, 233.1906)
  line L705 (353, 242.1906) -> (355, 243.3453)
  line L706 (368.75, 248.1084) -> (368.75, 250.4178)
  line L707 (346.75, 230.1084) -> (346.75, 232.4178)
  line L708 (359.25, 248.1084) -> (361.25, 246.9537)
  line L709 (355, 243.3453) -> (355, 245.6547)
  line L710 (360.5, 243.3453) -> (360.5, 245.6547)
  line L711 (383.25, 233.5725) -> (381.25, 232.4178)
  line L712 (364.75, 248.1084) -> (366.75, 246.9537)
  line L713 (352.25, 241.4178) -> (350.4572, 242.4529)
  line L714 (355, 243.3453) -> (355, 245.6547)
  line L715 (363.25, 248.1084) -> (363.25, 250.4178)
  line L716 (366.573, 251.4704) -> (364.75, 250.4178)
  line L717 (385.25, 232.4178) -> (383.25, 233.5725)
  line L718 (375.75, 239.1084) -> (377.75, 237.9537)
  line L719 (348.25, 232.4178) -> (348.25, 230.1084)
  line L720 (362, 245.6547) -> (362, 243.3453)
  line L721 (352.25, 241.4178) -> (350.4572, 242.4529)
  line L722 (362, 245.6547) -> (362, 243.3453)
  line L723 (355, 227.6547) -> (353, 228.8094)
  line L724 (347.5, 228.8094) -> (345.5, 227.6547)
  arc A17 (350.4572, 242.4529) -> (348.25, 240.0707) centre (375, 217.5) ccw
  line L725 (348.25, 232.4178) -> (348.25, 230.1084)
  line L726 (366.75, 246.9537) -> (368.75, 248.1084)
  line L727 (345.5, 227.6547) -> (345.5, 225.3453)
  line L728 (345.5, 227.6547) -> (345.5, 225.3453)
  line L729 (347.5, 237.8094) -> (345.8335, 236.8473)
  line L730 (350.25, 237.9537) -> (352.25, 239.1084)
  line L731 (355, 245.6547) -> (354.558, 245.9099)
  line L732 (352.25, 232.4178) -> (350.25, 233.5725)
  line L733 (344.75, 228.9537) -> (346.75, 230.1084)
  arc A18 (345.8335, 236.8473) -> (345.5, 236.3348) centre (375, 217.5) ccw
  line L734 (350.25, 233.5725) -> (348.25, 232.4178)
  line L735 (358.5, 246.8094) -> (356.5, 245.6547)
  line L736 (349.5, 236.6547) -> (347.5, 237.8094)
  line L737 (349.5, 225.3453) -> (349.5, 227.6547)
  line L738 (360.5, 245.6547) -> (358.5, 246.8094)
  line L739 (353, 237.8094) -> (351, 236.6547)
  line L740 (349.5, 236.6547) -> (347.5, 237.8094)
  line L741 (350.25, 224.5725) -> (348.25, 223.4178)
  line L742 (345.5, 225.3453) -> (347.5, 224.1906)
  line L743 (345.5, 236.3348) -> (345.5, 234.3453)
  line L744 (346.75, 232.4178) -> (344.75, 233.5725)
  line L745 (346.75, 232.4178) -> (344.75, 233.5725)
  line L746 (366, 245.6547) -> (364, 246.8094)
  line L747 (345.5, 225.3453) -> (347.5, 224.1906)
  line L748 (347.5, 224.1906) -> (349.5, 225.3453)
  line L749 (356.5, 245.6547) -> (356.5, 243.3453)
  line L750 (348.25, 239.1084) -> (350.25, 237.9537)
  line L751 (351, 227.6547) -> (351, 225.3453)
  line L752 (358.5, 242.1906) -> (360.5, 243.3453)
  line L753 (348.25, 239.1084) -> (350.25, 237.9537)
  line L754 (360.5, 245.6547) -> (358.5, 246.8094)
  line L755 (349.5, 234.3453) -> (349.5, 236.6547)
  arc A19 (366.8218, 251.5311) -> (366.573, 251.4704) centre (375, 217.5) ccw
  line L756 (350.25, 228.9537) -> (352.25, 230.1084)
  line L757 (349.5, 225.3453) -> (349.5, 227.6547)
  line L758 (355.75, 242.5725) -> (353.75, 241.4178)
  line L759 (350.25, 224.5725) -> (348.25, 223.4178)
  line L760 (345.5, 236.3348) -> (345.5, 234.3453)
  line L761 (347.5, 228.8094) -> (345.5, 227.6547)
  line L762 (353, 242.1906) -> (355, 243.3453)
  line L763 (368.3398, 251.8605) -> (369.5, 251.1906)
  line L764 (349.5, 227.6547) -> (347.5, 228.8094)
  line L765 (358.5, 242.1906) -> (360.5, 243.3453)
  line L766 (351, 236.6547) -> (351, 234.3453)
  line L767 (352.25, 223.4178) -> (350.25, 224.5725)
  line L768 (351, 225.3453) -> (353, 224.1906)
  line L769 (368.75, 250.4178) -> (366.8218, 251.5311)
  line L770 (351, 225.3453) -> (353, 224.1906)
  line L771 (347.5, 237.8094) -> (345.8335, 236.8473)
  line L772 (351, 234.3453) -> (353, 233.1906)
  line L773 (355.75, 242.5725) -> (353.75, 241.4178)
  line L774 (347.5, 233.1906) -> (349.5, 234.3453)
  arc A20 (345.8335, 236.8473) -> (345.5, 236.3348) centre (375, 217.5) ccw
  line L775 (345.5, 234.3453) -> (347.5, 233.1906)
  line L776 (351.2448, 243.2039) -> (353, 242.1906)
  line L777 (369.5, 246.8094) -> (367.5, 245.6547)
  line L778 (351.2448, 243.2039) -> (353, 242.1906)
  line L779 (361.25, 242.5725) -> (359.25, 241.4178)
  arc A21 (366.8218, 251.5311) -> (366.573, 251.4704) centre (375, 217.5) ccw
  line L780 (351, 236.6547) -> (351, 234.3453)
  line L781 (350.25, 233.5725) -> (348.25, 232.4178)
  line L782 (349.5, 227.6547) -> (347.5, 228.8094)
  line L783 (352.25, 232.4178) -> (350.25, 233.5725)
  line L784 (345.5, 234.3453) -> (347.5, 233.1906)
  line L785 (350.25, 237.9537) -> (352.25, 239.1084)
  line L786 (351, 234.3453) -> (353, 233.1906)
  line L787 (347.5, 233.1906) -> (349.5, 234.3453)
  line L788 (349.5, 234.3453) -> (349.5, 236.6547)
  line L789 (388, 218.6547) -> (386, 219.8094)
  line L790 (353.75, 214.4178) -> (353.75, 212.1084)
  line L791 (383.25, 228.9537) -> (385.25, 230.1084)
  line L792 (383.25, 224.5725) -> (381.25, 223.4178)
  line L793 (378.5, 209.6547) -> (378.5, 207.3453)
  line L794 (353.75, 221.1084) -> (355.75, 219.9537)
  line L795 (388.75, 246.9537) -> (390.75, 248.1084)
  line L796 (384, 243.3453) -> (386, 242.1906)
  line L797 (389.5, 216.3453) -> (391.5, 215.1906)
  line L798 (384, 245.6547) -> (384, 243.3453)
  line L799 (384, 216.3453) -> (386, 215.1906)
  line L800 (382.5, 207.3453) -> (382.5, 209.6547)
  line L801 (388.75, 215.5725) -> (386.75, 214.4178)
  line L802 (380.5, 206.1906) -> (382.5, 207.3453)
  line L803 (385.25, 223.4178) -> (383.25, 224.5725)
  line L804 (386.75, 214.4178) -> (386.75, 212.1084)
  line L805 (377.75, 206.5725) -> (375.75, 205.4178)
  line L806 (359.25, 214.4178) -> (359.25, 212.1084)
  line L807 (357.75, 212.1084) -> (357.75, 214.4178)
  line L808 (383.25, 228.9537) -> (385.25, 230.1084)
  line L809 (385.25, 223.4178) -> (383.25, 224.5725)
  line L810 (353.75, 214.4178) -> (353.75, 212.1084)
  line L811 (388, 243.3453) -> (388, 245.6547)
  line L812 (360.5, 225.3453) -> (360.5, 227.6547)
  line L813 (389.5, 243.3453) -> (391.5, 242.1906)
  line L814 (386.75, 250.4178) -> (386.75, 248.1084)
  line L815 (381.25, 230.1084) -> (383.25, 228.9537)
  line L816 (392.25, 232.4178) -> (392.25, 230.1084)
  line L817 (375.75, 212.1084) -> (377.75, 210.9537)
  line L818 (359.25, 214.4178) -> (359.25, 212.1084)
  line L819 (358.5, 224.1906) -> (360.5, 225.3453)
  line L820 (388, 245.6547) -> (386, 246.8094)
  line L821 (377.75, 210.9537) -> (379.75, 212.1084)
  line L822 (379.75, 205.4178) -> (377.75, 206.5725)
  line L823 (386, 219.8094) -> (384, 218.6547)
  line L824 (391.5, 219.8094) -> (389.5, 218.6547)
  line L825 (388, 216.3453) -> (388, 218.6547)
  line L826 (385.25, 212.1084) -> (385.25, 214.4178)
  line L827 (388, 216.3453) -> (388, 218.6547)
  line L828 (386.75, 248.1084) -> (388.75, 246.9537)
  line L829 (383.25, 224.5725) -> (381.25, 223.4178)
  line L830 (353.75, 230.1084) -> (355.75, 228.9537)
  line L831 (377, 207.3453) -> (377, 209.6547)
  line L832 (379.75, 248.1084) -> (379.75, 250.4178)
  line L833 (357.75, 212.1084) -> (357.75, 214.4178)
  line L834 (355.75, 228.9537) -> (357.75, 230.1084)
  line L835 (358.5, 228.8094) -> (356.5, 227.6547)
  line L836 (371.5, 245.6547) -> (369.5, 246.8094)
  line L837 (386, 215.1906) -> (388, 216.3453)
  line L838 (378.5, 207.3453) -> (380.5, 206.1906)
  line L839 (380.5, 210.8094) -> (378.5, 209.6547)
  line L840 (384, 243.3453) -> (386, 242.1906)
  line L841 (355, 225.3453) -> (355, 227.6547)
  line L842 (378.5, 227.6547) -> (378.5, 225.3453)
  line L843 (352.25, 239.1084) -> (352.25, 241.4178)
  line L844 (360.5, 227.6547) -> (358.5, 228.8094)
  line L845 (381.25, 230.1084) -> (383.25, 228.9537)
  line L846 (388, 243.3453) -> (388, 245.6547)
  line L847 (386, 242.1906) -> (388, 243.3453)
  line L848 (386, 219.8094) -> (384, 218.6547)
  line L849 (355.75, 224.5725) -> (353.75, 223.4178)
  line L850 (366.75, 219.9537) -> (368.75, 221.1084)
  line L851 (386.75, 214.4178) -> (386.75, 212.1084)
  line L852 (380.5, 206.1906) -> (382.5, 207.3453)
  line L853 (384, 218.6547) -> (384, 216.3453)
  line L854 (388.75, 215.5725) -> (386.75, 214.4178)
  line L855 (347.5, 206.1906) -> (349.5, 207.3453)
  line L856 (380.5, 219.8094) -> (378.5, 218.6547)
  line L857 (389.5, 236.6547) -> (389.5, 234.3453)
  line L858 (380.5, 210.8094) -> (378.5, 209.6547)
  line L859 (366, 216.3453) -> (366, 218.6547)
  line L860 (391.5, 219.8094) -> (389.5, 218.6547)
  line L861 (390.75, 230.1084) -> (390.75, 232.4178)
  line L862 (384, 245.6547) -> (384, 243.3453)
  line L863 (386, 246.8094) -> (384, 245.6547)
  line L864 (375.75, 232.4178) -> (375.75, 230.1084)
  line L865 (353, 206.1906) -> (355, 207.3453)
  line L866 (355.75, 224.5725) -> (353.75, 223.4178)
  line L867 (358.5, 228.8094) -> (356.5, 227.6547)
  line L868 (366.75, 215.5725) -> (364.75, 214.4178)
  line L869 (355, 209.6547) -> (353, 210.8094)
  line L870 (388.75, 246.9537) -> (390.75, 248.1084)
  line L871 (369.5, 224.1906) -> (371.5, 225.3453)
  line L872 (386, 242.1906) -> (388, 243.3453)
  line L873 (391.5, 246.8094) -> (389.5, 245.6547)
  line L874 (353.75, 241.4178) -> (353.75, 239.1084)
  line L875 (390.75, 241.4178) -> (388.75, 242.5725)
  line L876 (358.5, 224.1906) -> (360.5, 225.3453)
  line L877 (356.5, 227.6547) -> (356.5, 225.3453)
  line L878 (355, 225.3453) -> (355, 227.6547)
  line L879 (355, 218.6547) -> (353, 219.8094)
  line L880 (391.5, 246.8094) -> (389.5, 245.6547)
  line L881 (378.5, 209.6547) -> (378.5, 207.3453)
  line L882 (389.5, 218.6547) -> (389.5, 216.3453)
  line L883 (384, 218.6547) -> (384, 216.3453)
  line L884 (369.5, 219.8094) -> (367.5, 218.6547)
  line L885 (390.75, 214.4178) -> (388.75, 215.5725)
  line L886 (389.5, 245.6547) -> (389.5, 243.3453)
  line L887 (369.5, 219.8094) -> (367.5, 218.6547)
  line L888 (352.25, 205.4178) -> (350.25, 206.5725)
  line L889 (386, 215.1906) -> (388, 216.3453)
  line L890 (377.75, 210.9537) -> (379.75, 212.1084)
  line L891 (364, 215.1906) -> (366, 216.3453)
  line L892 (377, 216.3453) -> (377, 218.6547)
  line L893 (366.75, 219.9537) -> (368.75, 221.1084)
  line L894 (388.75, 242.5725) -> (386.75, 241.4178)
  line L895 (389.5, 216.3453) -> (391.5, 215.1906)
  line L896 (390.75, 241.4178) -> (388.75, 242.5725)
  line L897 (368.75, 214.4178) -> (366.75, 215.5725)
  line L898 (364.75, 221.1084) -> (366.75, 219.9537)
  line L899 (389.5, 218.6547) -> (389.5, 216.3453)
  line L900 (366, 218.6547) -> (364, 219.8094)
  line L901 (371.5, 245.6547) -> (369.5, 246.8094)
  line L902 (367.5, 218.6547) -> (367.5, 216.3453)
  line L903 (346.75, 212.1084) -> (346.75, 214.4178)
  line L904 (377.75, 215.5725) -> (375.75, 214.4178)
  line L905 (388, 218.6547) -> (386, 219.8094)
  line L906 (364, 215.1906) -> (366, 216.3453)
  line L907 (345.5, 209.6547) -> (345.5, 207.3453)
  line L908 (384, 236.6547) -> (384, 234.3453)
  line L909 (390.75, 214.4178) -> (388.75, 215.5725)
  line L910 (375.75, 214.4178) -> (375.75, 212.1084)
  line L911 (384, 216.3453) -> (386, 215.1906)
  line L912 (366, 216.3453) -> (366, 218.6547)
  line L913 (348.25, 212.1084) -> (350.25, 210.9537)
  line L914 (367.5, 236.6547) -> (367.5, 234.3453)
  line L915 (379.75, 214.4178) -> (377.75, 215.5725)
  line L916 (355.75, 237.9537) -> (357.75, 239.1084)
  line L917 (348.25, 240.0707) -> (348.25, 239.1084)
  line L918 (377.75, 246.9537) -> (379.75, 248.1084)
  line L919 (384, 236.6547) -> (384, 234.3453)
  line L920 (380.5, 219.8094) -> (378.5, 218.6547)
  line L921 (349.5, 209.6547) -> (347.5, 210.8094)
  line L922 (389.5, 236.6547) -> (389.5, 234.3453)
  line L923 (380.5, 215.1906) -> (382.5, 216.3453)
  line L924 (355, 234.3453) -> (355, 236.6547)
  line L925 (381.25, 214.4178) -> (381.25, 212.1084)
  line L926 (348.25, 214.4178) -> (348.25, 212.1084)
  line L927 (391.5, 237.8094) -> (389.5, 236.6547)
  line L928 (348.25, 214.4178) -> (348.25, 212.1084)
  line L929 (368.75, 214.4178) -> (366.75, 215.5725)
  line L930 (386.75, 250.4178) -> (386.75, 248.1084)
  line L931 (367.5, 218.6547) -> (367.5, 216.3453)
  line L932 (353, 210.8094) -> (351, 209.6547)
  line L933 (380.5, 215.1906) -> (382.5, 216.3453)
  line L934 (350.25, 206.5725) -> (348.25, 205.4178)
  line L935 (386, 233.1906) -> (388, 234.3453)
  line L936 (377.75, 215.5725) -> (375.75, 214.4178)
  line L937 (357.75, 232.4178) -> (355.75, 233.5725)
  line L938 (380.5, 242.1906) -> (382.5, 243.3453)
  line L939 (378.5, 216.3453) -> (380.5, 215.1906)
  line L940 (346.75, 212.1084) -> (346.75, 214.4178)
  line L941 (388, 234.3453) -> (388, 236.6547)
  line L942 (381.25, 214.4178) -> (381.25, 212.1084)
  line L943 (375.75, 214.4178) -> (375.75, 212.1084)
  line L944 (386, 237.8094) -> (384, 236.6547)
  line L945 (367.5, 216.3453) -> (369.5, 215.1906)
  line L946 (349.5, 209.6547) -> (347.5, 210.8094)
  line L947 (364.75, 221.1084) -> (366.75, 219.9537)
  line L948 (349.5, 207.3453) -> (349.5, 209.6547)
  line L949 (380.5, 246.8094) -> (378.5, 245.6547)
  line L950 (392.25, 232.4178) -> (392.25, 230.1084)
  line L951 (390.75, 248.1084) -> (390.75, 248.756)
  line L952 (357.75, 232.4178) -> (355.75, 233.5725)
  line L953 (366.75, 215.5725) -> (364.75, 214.4178)
  line L954 (367.5, 216.3453) -> (369.5, 215.1906)
  line L955 (382.5, 216.3453) -> (382.5, 218.6547)
  line L956 (375.75, 250.4178) -> (375.75, 248.1084)
  line L957 (353.75, 239.1084) -> (355.75, 237.9537)
  line L958 (366, 218.6547) -> (364, 219.8094)
  line L959 (346.75, 205.4178) -> (344.75, 206.5725)
  line L960 (344.75, 210.9537) -> (346.75, 212.1084)
  line L961 (356.5, 234.3453) -> (358.5, 233.1906)
  line L962 (390.75, 248.1084) -> (390.75, 248.756)
  line L963 (366, 234.3453) -> (366, 236.6547)
  line L964 (382.5, 218.6547) -> (380.5, 219.8094)
  line L965 (382.5, 218.6547) -> (380.5, 219.8094)
  line L966 (386, 237.8094) -> (384, 236.6547)
  line L967 (384, 234.3453) -> (386, 233.1906)
  line L968 (351, 207.3453) -> (353, 206.1906)
  line L969 (382.5, 243.3453) -> (382.5, 245.6547)
  line L970 (358.5, 233.1906) -> (360.5, 234.3453)
  line L971 (367.5, 236.6547) -> (367.5, 234.3453)
  line L972 (379.75, 214.4178) -> (377.75, 215.5725)
  line L973 (351, 209.6547) -> (351, 207.3453)
  line L974 (355.75, 233.5725) -> (353.75, 232.4178)
  line L975 (388.75, 233.5725) -> (386.75, 232.4178)
  line L976 (352.25, 212.1084) -> (352.25, 214.4178)
  line L977 (377, 216.3453) -> (377, 218.6547)
  arc A22 (390.75, 248.756) -> (386.8045, 250.4493) centre (375, 217.5) ccw
  line L978 (386.8045, 250.4493) -> (386.75, 250.4178)
  line L979 (351, 209.6547) -> (351, 207.3453)
  line L980 (347.5, 210.8094) -> (345.5, 209.6547)
  line L981 (349.5, 207.3453) -> (349.5, 209.6547)
  line L982 (366, 234.3453) -> (366, 236.6547)
  line L983 (377, 252.3453) -> (377, 252.4428)
  line L984 (355.75, 233.5725) -> (353.75, 232.4178)
  line L985 (345.5, 207.3453) -> (347.5, 206.1906)
  line L986 (379.75, 212.1084) -> (379.75, 214.4178)
  line L987 (351, 207.3453) -> (353, 206.1906)
  line L988 (361.25, 233.5725) -> (359.25, 232.4178)
  line L989 (385.25, 230.1084) -> (385.25, 232.4178)
  line L990 (386.75, 239.1084) -> (388.75, 237.9537)
  line L991 (344.75, 210.9537) -> (346.75, 212.1084)
  line L992 (378.5, 243.3453) -> (380.5, 242.1906)
  line L993 (378.5, 218.6547) -> (378.5, 216.3453)
  line L994 (379.75, 241.4178) -> (377.75, 242.5725)
  line L995 (359.25, 239.1084) -> (361.25, 237.9537)
  line L996 (377.75, 246.9537) -> (379.75, 248.1084)
  line L997 (367.5, 227.6547) -> (367.5, 225.3453)
  line L998 (379.75, 212.1084) -> (379.75, 214.4178)
  line L999 (352.25, 212.1084) -> (352.25, 214.4178)
  line L1000 (386.75, 239.1084) -> (388.75, 237.9537)